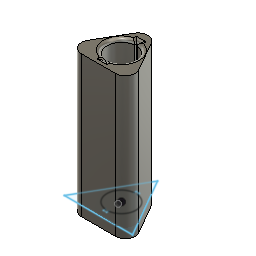
Xacto Cover (Autodesk Fusion 360 design; units mm, degrees)
Autodesk Fusion 360 part; units mm, degrees
sketch "Sketch1" plane through (0, 0, 0) normal (0, 1, 0) x (1, 0, 0)
  line L0 (-0.5, 5) -> (0.5, 5)
  line L1 (0.5, -5) -> (-0.5, -5)
  arc A0 (-0.5, 4.3715) -> (-0.5, -4.3715) centre (0, 0) ccw
  arc A1 (0.5, -4.3715) -> (0.5, 4.3715) centre (0, 0) ccw
  line L2 (0.5, 5) -> (0.5, 4.3715)
  line L3 (0.5, -4.3715) -> (0.5, -5)
  line L4 (-0.5, -5) -> (-0.5, -4.3715)
  line L5 (-0.5, 4.3715) -> (-0.5, 5)
  line L6 (10.3923, -7) -> (0, 11)
  line L7 (0, 11) -> (-10.3923, -7)
  line L8 (-10.3923, -7) -> (10.3923, -7)
  point P0 (0, -1)
  point P1 (0, -1)
  dimension "d1" = 8.8
  dimension "d10" = 1
  dimension "d11" = 6
  dimension "d12" = 4.4
  constraint coincident A0.centre A1.centre
  constraint perpendicular L0 L2
  constraint parallel L0 L1
  constraint parallel L2 L4
  constraint horizontal L0
  constraint coincident A0.start L4
  constraint coincident A1.start L2
  constraint concentric A0 A1
  constraint collinear L2 L3
  constraint collinear L4 L5
  constraint coincident P1 P0
  measures "d1" diameter of A0
  measures "d10" distance of A0.centre P0
  measures "d11" distance of P1 L8
  measures "d12" radius of A1
extrude "Extrude1" add sketch "Sketch1" along normal blind 40
extrude "Extrude2" add sketch "Sketch1" against normal blind 3 contours L0 L1 A0 A1 L2 L3 L4 L5 | L6 L7 L8
fillet "Fillet1" radius 1 curvature continuous 8 edges at (-4.4, 40, 0) (4.4, 40, 0) (-0.5, 40, -4.6857) (0.5, 40, -4.6857) (0, 40, -5) (-0.5, 40, 4.6857) (0, 40, 5) (0.5, 40, 4.6857)
fillet "Fillet2" radius 3 3 edges at (10.3923, 18.5, 7) (-10.3923, 18.5, 7) (0, 18.5, -11)
